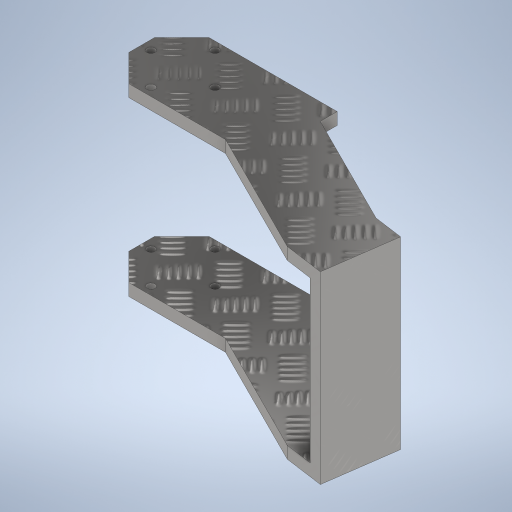
# Autodesk Inventor part: leg_part
Saved by Autodesk Inventor 2024 (Build 280153000, 153)
## iProperties
Created: 2024-02-16
Part Number: leg_part
Material: Generic
Document SubType Name: Modeling
Designer: kamil
Density: 1 g/cm^3
Appearance: Default
Author: kamil
Autodesk Inventor part; units mm, degrees
ref_plane "YZ Plane" through (0, 0, 0) normal (1, 0, 0) x (0, 1, 0)
ref_plane "XZ Plane" through (0, 0, 0) normal (0, 1, 0) x (-1, 0, 0)
ref_plane "XY Plane" through (0, 0, 0) normal (0, 0, 1) x (1, 0, 0)
sketch "Sketch1" plane through (0, 0, 0) normal (0, 1, 0) x (-1, 0, 0)
  line L0 (-20, 10) -> (12, 10)
  line L1 (20, 2) -> (20, -2)
  line L2 (12, -10) -> (-20, -10)
  line L3 (-20, -10) -> (-20, 10)
  line L4 (20, -10) -> (-20, 10) construction
  line L5 (20, 10) -> (-20, -10) construction
  line L6 (-12.1205, 10) -> (-20, -5.759)
  line L7 (-20, -5.759) -> (-50.8175, 9.6497)
  line L8 (-50.8175, 9.6497) -> (-42.9379, 25.4087)
  line L9 (-42.9379, 25.4087) -> (-12.1205, 10)
  line L10 (-42.9379, 25.4087) -> (-45.391, 7.8318)
  line L11 (-45.391, 7.8318) -> (-54.9943, 9.172)
  line L12 (-54.9943, 9.172) -> (-52.5413, 26.749)
  line L13 (-52.5413, 26.749) -> (-42.9379, 25.4087)
  line L14 (20, 4) -> (14, 10)
  line L15 (20, -4) -> (14, -10)
  line L16 (12, -10) -> (20, -2)
  line L17 (12, 10) -> (20, 2)
  line L18 (18.8, 3.2) -> (18.8, -3.2)
  point P0 (0, 0)
  point P1 (0, 0)
  point P2 (-47.8749, 8.1784)
  point P3 (20, 10)
  dimension "d0" = 40
  dimension "d1" = 20
  dimension "d2" = 6
  dimension "d3" = 6
  dimension "d4" = 6
  dimension "d5" = 6
  dimension "d11" = 161.38
  dimension "d32" = 8
  dimension "d33" = 8
  dimension "d34" = 8
  dimension "d35" = 8
  dimension "d43" = 1.2
  constraints: 38 end point, 16 point on line, 6 parallel, 3 perpendicular, 1 coincident, 1 horizontal, 1 midpoint, 1 vertical
  measures "d0" distance of L4.start L2.end
  measures "d1" distance of L5.start L4.start
  measures "d2" distance of L14.start L5.start
  measures "d3" distance of L14.end L5.start
  measures "d4" distance of L15.start L4.start
  measures "d5" distance of L15.end L4.start
  measures "d11" angle of L13 L9
  measures "d32" distance of L2.start point (20, -10)
  measures "d33" distance of L1.end point (20, -10)
  measures "d34" distance of L0.end point (20, 10)
  measures "d35" distance of L1.start point (20, 10)
  measures "d43" distance between parallel lines of L18 L1
extrude "Extrusion1" add sketch "Sketch1" along normal blind 3 contours L3 L7 L11 L10 L9 L0 | L0 L6 L3 | L0 L17 L18 L16 L2 L3 L6 | L10 L11 L7 L8 | L8 L7 L11 L12 L13
sketch "Sketch2" plane through (0, 0, 0) normal (0, -1, 0) x (1, 0, 0)
  line L0 (54.9943, 9.172) -> (47.8749, 8.1784) projected
  line L1 (54.9943, 9.172) -> (52.0231, 8.7573)
  line L2 (52.0231, 8.7573) -> (49.57, 26.3343)
  line L3 (49.57, 26.3343) -> (52.5413, 26.749)
  line L4 (52.5413, 26.749) -> (54.9943, 9.172)
  point P0 (0, 0)
  dimension "d8" = 3
  constraints: 8 end point, 2 parallel, 1 perpendicular, 1 point on line
  measures "d8" distance of L0.start L1.end
extrude "Extrusion2" add sketch "Sketch2" along normal blind 40
sketch "Sketch3" plane through (0, -40, 0) normal (0, -1, 0) x (1, 0, 0)
  line L0 (52.5413, 26.749) -> (54.9943, 9.172) projected
  line L1 (54.9943, 9.172) -> (52.5413, 26.749)
  line L2 (52.5413, 26.749) -> (42.9401, 25.409)
  line L3 (42.9401, 25.409) -> (45.3932, 7.8321)
  line L4 (45.3932, 7.8321) -> (54.9943, 9.172)
  line L5 (42.9401, 25.409) -> (12.1208, 9.9994)
  line L6 (12.1208, 9.9994) -> (20, -5.759)
  line L7 (20, -5.759) -> (50.8193, 9.6506)
  line L8 (50.8193, 9.6506) -> (42.9401, 25.409)
  line L9 (47.8749, 8.1784) -> (20, -5.759) projected
  line L10 (20, -5.759) -> (20, -10) projected
  line L11 (20, -10) -> (20, 9.9994)
  line L12 (20, 9.9994) -> (-12, 9.9994)
  line L13 (-20, 1.9994) -> (-20, -2)
  line L14 (-12, -10) -> (20, -10)
  line L15 (-20, -4) -> (-14, -10)
  line L16 (-20, 3.9994) -> (-14, 9.9994)
  line L17 (-20, 1.9994) -> (-12, 9.9994)
  line L18 (-20, -2) -> (-12, -10)
  line L19 (-18.8, -3.2) -> (-18.8, 3.1994)
  point P0 (0, 0)
  point P1 (-20, 9.9994)
  point P2 (-20, -10)
  point P3 (47.8749, 8.1784)
  point P4 (-20, 9.9994)
  point P5 (-20, -10)
  point P6 (20, -5.759)
  point P7 (20, -5.759)
  point P8 (-18.8, 3.2)
  dimension "d12" = 40
  dimension "d13" = 6
  dimension "d14" = 6
  dimension "d15" = 6
  dimension "d16" = 6
  dimension "d28" = 8
  dimension "d29" = 8
  dimension "d30" = 8
  dimension "d31" = 8
  dimension "d45" = 1.2
  constraints: 34 end point, 14 point on line, 7 parallel, 3 perpendicular, 2 collinear, 1 vertical
  measures "d12" distance of point (-20, 9.999) L11.end
  measures "d13" distance of L15.start point (-20, -10)
  measures "d14" distance of L15.end point (-20, -10)
  measures "d15" distance of L16.start point (-20, 9.999)
  measures "d16" distance of L16.end point (-20, 9.999)
  measures "d28" distance of L13.start point (-20, 9.999)
  measures "d29" distance of L12.end point (-20, 9.999)
  measures "d30" distance of L13.end point (-20, -10)
  measures "d31" distance of L14.start point (-20, -10)
  measures "d45" distance between parallel lines of L19 L13
extrude "Extrusion3" add sketch "Sketch3" along normal blind 3 contours L0 L4 L7 L8 L2 | L8 L7 L4 L3 | L3 L4 L7 L11 L12 L5 | L12 L11 L6 | L6 L10 L14 L18 L19 L17 L12
sketch "Sketch4" plane through (0, 3, 0) normal (0, 1, 0) x (1, 0, 0)
  line L0 (-20, -1.9994) -> (-20, 2) projected
  line L1 (-20, 0.0003) -> (-8.5, 0.0003)
  circle A0 centre (-0.5, 0.0003) radius 1
  circle A1 centre (-8.5, 8.0003) radius 1
  circle A2 centre (-16.5, 0.0003) radius 1
  circle A3 centre (-8.5, -7.9997) radius 1
  point P0 (0, 0)
  point P1 (-20, -3.9994)
  point P2 (-20, 4)
  dimension "d19" = 11.5
  dimension "d20" = 2
  dimension "d21" = 8
  dimension "d24" = 360
  constraints: 4 centre point, 2 end point, 1 horizontal, 1 midpoint, 9 other
  measures "d19" distance of L1.start L1.end
  measures "d20" diameter of A0
  measures "d21" distance of A0.centre L1.end
extrude "Extrusion4" cut sketch "Sketch4" against normal blind 50
equation "\"d3\" = d2"
equation "\"d4\" = d2"
equation "\"d5\" = d4"
equation "\"d33\" = d32"
equation "\"d34\" = d32"
equation "\"d35\" = d34"
equation "\"d14\" = d13"
equation "\"d15\" = d13"
equation "\"d16\" = d15"
equation "\"d29\" = d28"
equation "\"d30\" = d28"
equation "\"d31\" = d30"
body "Solid1"
